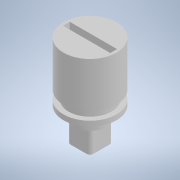
# Autodesk Inventor part: lock_insert_na
Saved by Autodesk Inventor 2021 (Build 250183000, 183)
## iProperties
Created: 2025-08-10
Part Number: lock_insert_na
Material: Generic
Catalog Web Link: www.cadenas.de
Description: LOCK INSERT-WALLMOUNT
Vendor: RITTAL
Document SubType Name: Modeling
Designer: psAdmin
Manufacturer: RITTAL
Mass: 3.5301 g
Surface Area: 18.017 cm^2
Volume: 3.5301 cm^3
Density: 1 g/cm^3
Appearance: PSOLRGB-175-175-175
Category: PARTsolutions
Company: RITTAL
Title: lock_insert_na
Author: Cadenas PARTsolutions
Comments: WALLMOUNT
PSOL_IDENT_0: {$CADENAS_DATA/23d-libs/rittal/rittal_north_america/enclosure_systems/compact_enclosures/wm_parts/wm
PSOL_IDENT_1: _one_door_parts/lock_insert.prj},173 {VTYP=3D},{NB=lock_insert_na},{LINA=lock_insert_na},{NN=LOCK IN
PSOL_IDENT_2: SERT},{DATE=20.08.2024 09:24:21},{GEOMDATE=25.11.2019 11:27:25},{VERSION=},{LINEID=10},{WBVAR=},{WBN
PSOL_IDENT_3: UMERIC=}  {NB=lock_insert_na},{LINA=lock_insert_na},{KT=DUMMY},{PN=lock_insert},{DETAIL=MIN}
NB: lock_insert_na
NN: LOCK INSERT
NT: WALLMOUNT
NBSYN: $PN._na
LINA: lock_insert_na
CATALOG: Rittal
PN: lock_insert
DETAIL: 0
SUPPLIER: RITTAL
ARTICLENO: lock_insert_na
BOMINFO: lock_insert_na
CREATOR: CADENAS GmbH
Autodesk Inventor part; units mm, degrees
sketch "Sketch_1" plane through (0, 0, 0) normal (0, 0, 1) x (1, 0, 0)
  line L0 (0, -20.5) -> (0, 0)
  line L1 (0, 0) -> (7.85, 0)
  line L2 (7.85, 0) -> (7.85, -13.35)
  line L3 (7.85, -13.35) -> (6.375, -13.35)
  line L4 (6.375, -13.35) -> (6.375, -15.85)
  line L5 (6.375, -15.85) -> (7.85, -15.85)
  line L6 (7.85, -15.85) -> (7.85, -17.35)
  line L7 (7.85, -17.35) -> (4.925, -17.35)
  line L8 (4.925, -17.35) -> (4.925, -20.5)
  line L9 (4.925, -20.5) -> (0, -20.5)
  line L10 (0, -20.5) -> (0, 0)
  constraints: 22 end point
revolve "Revolution1" add sketch "Sketch_1" angle 360 about axis through (0, -20.5, 0) along (0, -1, 0)
sketch "Sketch_2" plane through (0, -20.5, 0) normal (0, 1, 0) x (1, 0, 0)
  arc A0 (-3.4, -2.4) -> (-2.4, -3.4) centre (-2.4, -2.4) ccw
  line L0 (-2.4, -3.4) -> (2.4, -3.4)
  arc A1 (2.4, -3.4) -> (3.4, -2.4) centre (2.4, -2.4) ccw
  line L1 (3.4, -2.4) -> (3.4, 2.4)
  arc A2 (3.4, 2.4) -> (2.4, 3.4) centre (2.4, 2.4) ccw
  line L2 (2.4, 3.4) -> (-2.4, 3.4)
  arc A3 (-2.4, 3.4) -> (-3.4, 2.4) centre (-2.4, 2.4) ccw
  line L3 (-3.4, 2.4) -> (-3.4, -2.4)
  circle A4 centre (0, 0) radius 2.455
  constraints: 8 end point, 8 point on circle, 5 centre point
extrude "Extrusion1" add sketch "Sketch_2" against normal blind 6.5
sketch "Sketch_3" plane through (0, 0, 0) normal (0, 1, 0) x (-1, 0, 0)
  line L0 (7, -1) -> (7, 1)
  line L1 (7, 1) -> (-7, 1)
  line L2 (-7, 1) -> (-7, -1)
  line L3 (-7, -1) -> (7, -1)
  constraints: 8 end point
extrude "Extrusion2" cut sketch "Sketch_3" against normal blind 2.71
ref_plane "insert_to_lock_XY" through (0, 0, 0) normal (0, 1, 0) x (1, 0, 0)
ref_plane "insert_to_lock_YZ" through (0, 0, 0) normal (1, 0, 0) x (0, 0, -1)
ref_plane "insert_to_lock_ZX" through (0, 0, 0) normal (0, 0, -1) x (0, 1, 0)
body "Solid1"
